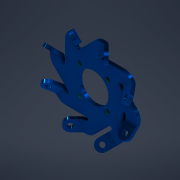
# Autodesk Inventor part: frame
Saved by Autodesk Inventor 2021.3 (Build 253353000, 353)
## iProperties
Created: 2021-10-17
Part Number: frame
Material: Stainless Steel, Polished
Document SubType Name: Sheet Metal
Designer: ASUS
Density: 8 g/cm^3
Sheet Metal Rule: Default_mm
Appearance: Stainless - Polished
Author: ASUS
Autodesk Inventor part; units mm, degrees
ref_plane "YZ Plane" through (0, 0, 0) normal (1, 0, 0) x (0, 1, 0)
ref_plane "XZ Plane" through (0, 0, 0) normal (0, 1, 0) x (-1, 0, 0)
ref_plane "XY Plane" through (0, 0, 0) normal (0, 0, 1) x (1, 0, 0)
sketch "Sketch1" plane through (0, 0, 0) normal (0, 0, 1) x (1, 0, 0)
  circle A0 centre (0, 0) radius 9
  circle A1 centre (0, 0) radius 30
  circle A2 centre (12.5, 23) radius 1.5
  line L0 (12.5, 19.5) -> (4.5, 19.5)
  line L1 (12.5, 17.5) -> (4.5, 17.5)
  arc A3 (4.5, 19.5) -> (4.5, 17.5) centre (4.5, 18.5) ccw
  arc A4 (12.5, 19.5) -> (12.5, 26.5) centre (12.5, 23) ccw
  line L2 (12.5, 26.5) -> (4.5, 26.5)
  circle A5 centre (-7.4246, 25.1023) radius 1.5
  line L3 (-4.9497, 22.6274) -> (-10.6066, 16.9706)
  line L4 (-3.5355, 21.2132) -> (-9.1924, 15.5563)
  arc A6 (-10.6066, 16.9706) -> (-9.1924, 15.5563) centre (-9.8995, 16.2635) ccw
  arc A7 (-4.9497, 22.6274) -> (-9.8995, 27.5772) centre (-7.4246, 25.1023) ccw
  line L5 (-9.8995, 27.5772) -> (-15.5563, 21.9203)
  circle A8 centre (-23, 12.5) radius 1.5
  line L6 (-19.5, 12.5) -> (-19.5, 4.5)
  line L7 (-17.5, 12.5) -> (-17.5, 4.5)
  arc A9 (-19.5, 4.5) -> (-17.5, 4.5) centre (-18.5, 4.5) ccw
  arc A10 (-19.5, 12.5) -> (-26.5, 12.5) centre (-23, 12.5) ccw
  line L8 (-26.5, 12.5) -> (-26.5, 4.5)
  circle A11 centre (-25.1023, -7.4246) radius 1.5
  line L9 (-22.6274, -4.9497) -> (-16.9706, -10.6066)
  line L10 (-21.2132, -3.5355) -> (-15.5563, -9.1924)
  arc A12 (-16.9706, -10.6066) -> (-15.5563, -9.1924) centre (-16.2635, -9.8995) ccw
  arc A13 (-22.6274, -4.9497) -> (-27.5772, -9.8995) centre (-25.1023, -7.4246) ccw
  line L11 (-27.5772, -9.8995) -> (-21.9203, -15.5563)
  circle A14 centre (-12.5, -23) radius 1.5
  line L12 (-12.5, -19.5) -> (-4.5, -19.5)
  line L13 (-12.5, -17.5) -> (-4.5, -17.5)
  arc A15 (-4.5, -19.5) -> (-4.5, -17.5) centre (-4.5, -18.5) ccw
  arc A16 (-12.5, -19.5) -> (-12.5, -26.5) centre (-12.5, -23) ccw
  line L14 (-12.5, -26.5) -> (-4.5, -26.5)
  circle A17 centre (7.4246, -25.1023) radius 1.5
  line L15 (4.9497, -22.6274) -> (10.6066, -16.9706)
  line L16 (3.5355, -21.2132) -> (9.1924, -15.5563)
  arc A18 (10.6066, -16.9706) -> (9.1924, -15.5563) centre (9.8995, -16.2635) ccw
  arc A19 (4.9497, -22.6274) -> (9.8995, -27.5772) centre (7.4246, -25.1023) ccw
  line L17 (9.8995, -27.5772) -> (15.5563, -21.9203)
  circle A20 centre (23, -12.5) radius 1.5
  line L18 (19.5, -12.5) -> (19.5, -4.5)
  line L19 (17.5, -12.5) -> (17.5, -4.5)
  arc A21 (19.5, -4.5) -> (17.5, -4.5) centre (18.5, -4.5) ccw
  arc A22 (19.5, -12.5) -> (26.5, -12.5) centre (23, -12.5) ccw
  line L20 (26.5, -12.5) -> (26.5, -4.5)
  circle A23 centre (25.1023, 7.4246) radius 1.5
  line L21 (22.6274, 4.9497) -> (16.9706, 10.6066)
  line L22 (21.2132, 3.5355) -> (15.5563, 9.1924)
  arc A24 (16.9706, 10.6066) -> (15.5563, 9.1924) centre (16.2635, 9.8995) ccw
  arc A25 (22.6274, 4.9497) -> (27.5772, 9.8995) centre (25.1023, 7.4246) ccw
  line L23 (27.5772, 9.8995) -> (21.9203, 15.5563)
  line L24 (-3.5355, 21.2132) -> (-0.299, 24.4497)
  line L25 (4.6508, 26.5) -> (4.5, 26.5)
  arc A26 (4.6508, 26.5) -> (-0.299, 24.4497) centre (4.6508, 19.5) ccw
  line L26 (-17.5, 12.5) -> (-17.5, 17.0772)
  arc A27 (-15.4497, 22.0269) -> (-17.5, 17.0772) centre (-10.5, 17.0772) ccw
  line L27 (-21.2132, -3.5355) -> (-24.4497, -0.299)
  arc A28 (-26.5, 4.6508) -> (-24.4497, -0.299) centre (-19.5, 4.6508) ccw
  line L28 (-12.5, -17.5) -> (-17.0772, -17.5)
  arc A29 (-22.0269, -15.4497) -> (-17.0772, -17.5) centre (-17.0772, -10.5) ccw
  line L29 (3.5355, -21.2132) -> (0.299, -24.4497)
  arc A30 (-4.6508, -26.5) -> (0.299, -24.4497) centre (-4.6508, -19.5) ccw
  line L30 (17.5, -12.5) -> (17.5, -17.0772)
  arc A31 (15.4497, -22.0269) -> (17.5, -17.0772) centre (10.5, -17.0772) ccw
  line L31 (21.2132, 3.5355) -> (24.4497, 0.299)
  arc A32 (26.5, -4.6508) -> (24.4497, 0.299) centre (19.5, -4.6508) ccw
  line L32 (12.5, 17.5) -> (17.0772, 17.5)
  arc A33 (22.0269, 15.4497) -> (17.0772, 17.5) centre (17.0772, 10.5) ccw
  line L33 (0, 0) -> (8.4853, 8.4853) construction
  line L34 (0, 0) -> (12, 0) construction
  circle A34 centre (8.4853, 8.4853) radius 1.5075
  circle A35 centre (-8.4853, 8.4853) radius 1.5075
  circle A36 centre (-8.4853, -8.4853) radius 1.5075
  circle A37 centre (8.4853, -8.4853) radius 1.5075
  point P0 (-15.4497, 22.0269)
  dimension "d0" = 18
  dimension "d1" = 60
  dimension "d2" = 3
  dimension "d5" = 8
  dimension "d6" = 2
  dimension "d10" = 360
  dimension "d12" = 7
  dimension "d15" = 360
  dimension "d17" = 3.5
  dimension "d18" = 12
  dimension "d19" = 45
  dimension "d20" = 3.015
  dimension "d23" = 360
  constraints: 70 end point, 48 point on circle, 38 centre point, 11 coincident, 4 horizontal, 2 tangent, 1 equal length, 1 parallel, 179 other
  measures "d0" diameter of A0
  measures "d1" diameter of A1
  measures "d2" diameter of A2
  measures "d5" distance of L0.start L0.end
  measures "d6" distance between parallel lines of L0 L1
  measures "d12" radius of A26
  measures "d17" distance of L2.start A2.centre
  measures "d18" distance of L33.start L33.end
  measures "d19" angle of L34 L33
  measures "d20" diameter of A34
extrude "Extrusion1" add sketch "Sketch1" along normal mid plane 2 contours L0 A3 L1 L32 A33 L23 A25 L21 A24 L22 L31 A32 L20 A22 L18 A21 L19 L30 A31 L17 A19 L15 A18 L16 L29 A30 L14 A16 L12 A15 L13 L28 A29 L11 A13 L9 A12 L10 L27 A28 L8 A10 L6 A9 L7 L26 A27 L5 A7 L3 A6 L4 L24 A26 L2 A4
sketch "Sketch2" plane through (0, 0, 1) normal (0, 0, 1) x (1, 0, 0)
  line L0 (12.5, 26.5) -> (4.6508, 26.5) projected
  line L1 (6.55, 26.5) -> (6.55, 19.5)
  line L2 (4.5, 19.5) -> (12.5, 19.5) projected
  point P0 (0, 0)
  constraints: 2 end point, 2 point on line, 1 vertical
fold "Fold1" angle 45 bend radius 2 thickness 2 k factor 0.44 line from (6.55, 26.5, 1) to (6.55, 19.5, 1) line at bend centre moving side (1, 0, 0) folds toward (0, 0, 1)
pattern_circular "Circular Pattern1" count 8 over 360 about axis through (0, 0, 0) along (0, 0, 1) of "Fold1"
thread "Thread1" size "M3x0.5" class "6H" standard "ANSI Metric M Profile" full length
thread "Thread2" size "M3x0.5" class "6H" standard "ANSI Metric M Profile" full length
thread "Thread3" size "M3x0.5" class "6H" standard "ANSI Metric M Profile" full length
thread "Thread4" size "M3x0.5" class "6H" standard "ANSI Metric M Profile" full length
equation "\"d27\" = Thickness"
equation "\"d28\" = BendReliefWidth"
equation "\"d29\" = BendReliefDepth"
equation "\"d30\" = MinimumRemnant"
equation "\"d31\" = TransitionRadius"
equation "\"d33\" = BendRadius"
equation "\"BendRadius\" = Thickness"
equation "\"BendReliefWidth\" = Thickness"
equation "\"BendReliefDepth\" = 0.5 * Thickness"
equation "\"CornerReliefSize\" = 4 * Thickness"
equation "\"MinimumRemnant\" = 2 * Thickness"
equation "\"TransitionRadius\" = BendRadius"
equation "\"JacobiRadiusSize\" = BendRadius"
equation "\"GapSize\" = Thickness"
equation "\"Thickness\" = 2"
body "Solid1"
